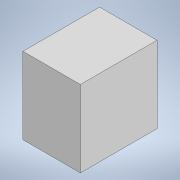
# Autodesk Inventor part: Goal
Saved by Autodesk Inventor 2021 (Build 250183000, 183)
## iProperties
Created: 2022-07-02
Part Number: Goal
Material: 一般
Document SubType Name: Modeling
Designer: tazak
Density: 1 g/cm^3
Appearance: 既定
Author: tazak
Autodesk Inventor part; units mm, degrees
ref_plane "YZ Plane" through (0, 0, 0) normal (1, 0, 0) x (0, 1, 0)
ref_plane "XZ Plane" through (0, 0, 0) normal (0, 1, 0) x (-1, 0, 0)
ref_plane "XY Plane" through (0, 0, 0) normal (0, 0, 1) x (1, 0, 0)
sketch "スケッチ1" plane through (0, 0, 0) normal (0, 0, 1) x (1, 0, 0)
  line L0 (12000, 2000) -> (13500, 2000)
  line L1 (13500, 2000) -> (13500, 0)
  line L2 (13500, 0) -> (12000, 0)
  line L3 (12000, 0) -> (12000, 2000)
  point P0 (0, 0)
  dimension "d13" = 1500
  dimension "d23" = 2000
  dimension "d24" = 12000
  dimension "d28" = 0
  constraints: 8 end point, 2 parallel, 1 horizontal, 1 perpendicular
  measures "d13" distance of L0.start L0.end
  measures "d23" distance of L2.end L0.start
  measures "d24" distance from line of L3 point (0, 0)
  measures "d28" distance from line of point (0, 0) L2
extrude "押し出し1" add sketch "スケッチ1" along normal blind 2000
